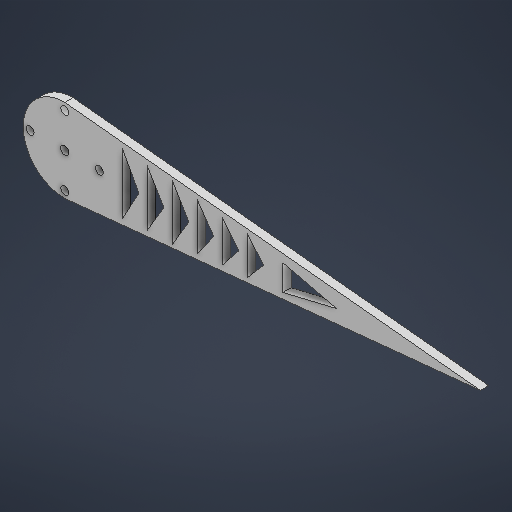
# Autodesk Inventor part: link2
Saved by Autodesk Inventor 2026.1 (Build 301233020, 233B)
## iProperties
Created: 2026-04-17
Part Number: link2
Material: Generic
Document SubType Name: Modeling
Designer: kadir
Density: 1 g/cm^3
Appearance: Default
Author: kadir
Autodesk Inventor part; units mm, degrees
ref_plane "YZ Plane" through (0, 0, 0) normal (1, 0, 0) x (0, 1, 0)
ref_plane "XZ Plane" through (0, 0, 0) normal (0, 1, 0) x (-1, 0, 0)
ref_plane "XY Plane" through (0, 0, 0) normal (0, 0, 1) x (1, 0, 0)
sketch "Sketch1" plane through (0, 0, 0) normal (0, 0, 1) x (1, 0, 0)
  circle A0 centre (0, 0) radius 15
  circle A1 centre (-12.5, 0) radius 1.4
  circle A2 centre (0, -12.5) radius 1.4
  circle A3 centre (12.5, 0) radius 1.4
  circle A4 centre (0, 12.5) radius 1.4
  arc A5 (139.8092, 1.0191) -> (139.8092, -1.0191) centre (150, 0) ccw
  line L0 (0, 15) -> (150, 0)
  line L1 (0, -15) -> (150, 0)
  line L2 (29.7634, 10.0809) -> (35.7634, 10.0809)
  line L3 (35.7634, 10.0809) -> (35.7634, -10.0809)
  line L4 (35.7634, -10.0809) -> (29.7634, -10.0809)
  line L5 (29.7634, -10.0809) -> (29.7634, 10.0809)
  line L6 (29.7634, 10.0809) -> (35.7634, -10.0809) construction
  line L7 (35.7634, 10.0809) -> (29.7634, -10.0809) construction
  line L8 (38.7634, 10.0809) -> (44.7634, 10.0809)
  line L9 (44.7634, 10.0809) -> (44.7634, -10.0809)
  line L10 (44.7634, -10.0809) -> (38.7634, -10.0809)
  line L11 (38.7634, -10.0809) -> (38.7634, 10.0809)
  line L12 (38.7634, 10.0809) -> (44.7634, -10.0809) construction
  line L13 (44.7634, 10.0809) -> (38.7634, -10.0809) construction
  line L14 (47.7634, 8.546) -> (53.7634, 8.546)
  line L15 (53.7634, 8.546) -> (53.7634, -8.546)
  line L16 (53.7634, -8.546) -> (47.7634, -8.546)
  line L17 (47.7634, -8.546) -> (47.7634, 8.546)
  line L18 (47.7634, 8.546) -> (53.7634, -8.546) construction
  line L19 (53.7634, 8.546) -> (47.7634, -8.546) construction
  line L20 (62.7634, 7.5) -> (56.7634, 7.5)
  line L21 (56.7634, 7.5) -> (56.7634, -7.5)
  line L22 (56.7634, -7.5) -> (62.7634, -7.5)
  line L23 (62.7634, -7.5) -> (62.7634, 7.5)
  line L24 (62.7634, 7.5) -> (56.7634, -7.5) construction
  line L25 (56.7634, 7.5) -> (62.7634, -7.5) construction
  line L26 (71.7634, 6.9773) -> (65.7634, 6.9773)
  line L27 (65.7634, 6.9773) -> (65.7634, -6.9773)
  line L28 (65.7634, -6.9773) -> (71.7634, -6.9773)
  line L29 (71.7634, -6.9773) -> (71.7634, 6.9773)
  line L30 (71.7634, 6.9773) -> (65.7634, -6.9773) construction
  line L31 (65.7634, 6.9773) -> (71.7634, -6.9773) construction
  line L32 (20.7634, 11) -> (26.7634, 11)
  line L33 (26.7634, 11) -> (26.7634, -11)
  line L34 (26.7634, -11) -> (20.7634, -11)
  line L35 (20.7634, -11) -> (20.7634, 11)
  line L36 (20.7634, 11) -> (26.7634, -11) construction
  line L37 (26.7634, 11) -> (20.7634, -11) construction
  line L38 (20.7634, 11) -> (26.7634, 0)
  line L39 (20.7634, -11) -> (26.7634, 0)
  line L40 (29.7634, 10.0809) -> (35.7634, 0)
  line L41 (29.7634, -10.0809) -> (35.7634, 0)
  line L42 (38.7634, 10.0809) -> (44.7634, 0)
  line L43 (38.7634, -10.0809) -> (44.7634, 0)
  line L44 (47.7634, 8.546) -> (53.7634, 0)
  line L45 (47.7634, -8.546) -> (53.7634, 0)
  line L46 (56.7634, 7.5) -> (62.7634, 0)
  line L47 (56.7634, -7.5) -> (62.7634, 0)
  line L48 (65.7634, 6.9773) -> (71.7634, 0)
  line L49 (65.7634, -6.9773) -> (71.7634, 0)
  line L50 (78.7015, 4.273) -> (78.7015, -5.0405)
  line L51 (78.7015, -5.0405) -> (98.1361, -0.3837)
  line L52 (98.1361, -0.3837) -> (78.7015, 4.273)
  point P0 (32.7634, 0)
  point P1 (41.7634, 0)
  point P2 (50.7634, 0)
  point P3 (59.7634, 0)
  point P4 (68.7634, 0)
  point P5 (23.7634, 0)
  dimension "d0" = 30
  dimension "d1" = 2.8
  dimension "d2" = 12.5
  dimension "d5" = 360
  dimension "d7" = 150
  dimension "d8" = 9
  dimension "d9" = 9
  dimension "d10" = 9
  dimension "d11" = 9
  dimension "d12" = 6
  dimension "d13" = 6
  dimension "d14" = 6
  dimension "d15" = 6
  dimension "d16" = 6
  dimension "d17" = 6
  dimension "d18" = 9
  dimension "d19" = 22
  constraints: 106 end point, 18 midpoint, 13 parallel, 6 centre point, 6 horizontal, 6 horizontal alignment, 6 perpendicular, 4 point on circle, 2 point on line, 1 coincident, 1 vertical, 9 other
  measures "d0" diameter of A0
  measures "d1" diameter of A1
  measures "d2" distance of point (0, 0) A1.centre
  measures "d7" distance of L0.end point (0, 0)
  measures "d8" distance of point (41.763, 0) point (32.763, 0)
  measures "d9" distance of point (50.763, 0) point (41.763, 0)
  measures "d10" distance of point (50.763, 0) point (59.763, 0)
  measures "d11" distance of point (68.763, 0) point (59.763, 0)
  measures "d12" distance of L26.start L26.end
  measures "d13" distance of L20.start L20.end
  measures "d14" distance of L14.start L14.end
  measures "d15" distance of L8.start L8.end
  measures "d16" distance of L2.start L2.end
  measures "d17" distance of L33.end L34.end
  measures "d18" distance of point (32.763, 0) point (23.763, 0)
  measures "d19" distance of L34.end L32.start
extrude "Extrusion1" add sketch "Sketch1" along normal blind 3 contours L0 A0 L1 | L0 A5 L1 A0 | L0 L1 A5 | L2 L3 L40 | L41 L3 L4 | L8 L9 L42 | L43 L9 L10 | L14 L15 L44 | L45 L15 L16 | L23 L46 L20 | L23 L22 L47 | L29 L48 L26 | L29 L28 L49 | L32 L33 L38 | L39 L33 L34
sketch "Sketch2" plane through (0, 0, 3) normal (0, 0, 1) x (1, 0, 0)
  circle A0 centre (0, 0) radius 1.5
  dimension "d22" = 3
  constraints: 1 centre point, 1 coincident
  measures "d22" diameter of A0
extrude "Extrusion2" cut sketch "Sketch2" against normal through all
body "Solid1"
